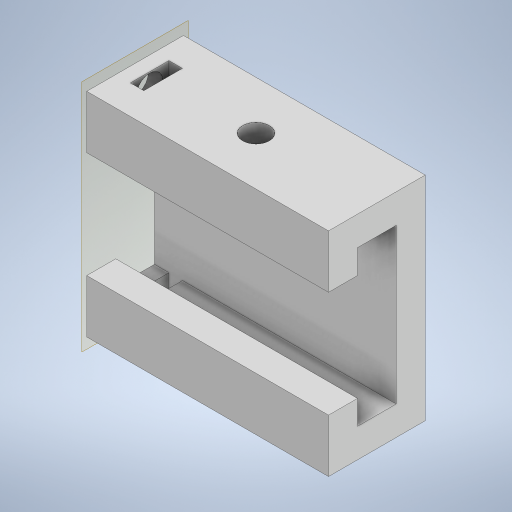
# Autodesk Inventor part: cuerpo_obj2
Saved by Autodesk Inventor 2023.2 (Build 272271030, 271C)
## iProperties
Created: 2023-02-25
Part Number: cuerpo_obj2
Material: Generic
Document SubType Name: Modeling
Designer: Cris Pat
Density: 1 g/cm^3
Appearance: Default
Author: Cris Pat
Autodesk Inventor part; units mm, degrees
ref_plane "XY Plane" through (0, 0, 0) normal (0, 0, 1) x (1, 0, 0)
sketch "Sketch1" plane through (0, 0, 0) normal (1, 0, 0) x (0, 1, 0)
  line L0 (11, 10) -> (11, 4)
  line L1 (11, 4) -> (16, 4)
  line L2 (16, 4) -> (16, -4)
  line L3 (16, -4) -> (-16, -4)
  line L4 (-16, -4) -> (-16, 4)
  line L5 (-16, 4) -> (-11, 4)
  line L6 (-11, 4) -> (-11, 10)
  line L7 (-11, 10) -> (-22, 10)
  line L8 (-22, 10) -> (-22, -10)
  line L9 (-22, -10) -> (22, -10)
  line L10 (22, -10) -> (22, 10)
  line L11 (22, 10) -> (11, 10)
  line L12 (11, 7) -> (-11, 7) construction
  line L13 (16, 0) -> (-16, 0) construction
  point P0 (0, 0)
  point P1 (-13.5, 4)
  point P2 (13.5, 4)
  point P3 (16.5, 10)
  point P4 (-16.5, 10)
  point P5 (22, 0)
  point P6 (0, -10)
  point P7 (0, 7)
  point P8 (0, 0)
  dimension "d0" = 22
  dimension "d1" = 32
  dimension "d2" = 6
  dimension "d3" = 14
  dimension "d4" = 44
  dimension "d5" = 20
  constraints: 28 end point, 12 midpoint, 10 perpendicular, 3 horizontal alignment, 3 point on line, 2 vertical alignment, 1 coincident, 1 vertical
  measures "d0" distance between parallel lines of L6 L0
  measures "d1" distance from line of L4 L13.start
  measures "d2" distance from line of point (-13.5, 4) L7
  measures "d3" distance between parallel lines of L7 L3
  measures "d4" distance between parallel lines of L8 L10
  measures "d5" distance between parallel lines of L7 L9
extrude "Extrusion1" add sketch "Sketch1" along normal mid plane 50
ref_plane "Work Plane1" through (0, 22, 0) normal (0, 1, 0) x (-1, 0, 0)
sketch "Sketch2" plane through (0, 22, 0) normal (0, 1, 0) x (-1, 0, 0)
  line L0 (25, 10) -> (-25, 10) construction
  line L1 (-25, -10) -> (-25, 10) construction
  line L2 (25, -10) -> (-25, -10) construction
  line L3 (25, 10) -> (25, -10) construction
  line L4 (-25, 0) -> (25, 0) construction
  circle A0 centre (0, 0) radius 2.75
  point P0 (0, 0)
  dimension "d9" = 5.5
  dimension "d10" = 25
  constraints: 3 midpoint, 2 end point, 1 centre point
  measures "d9" diameter of A0
  measures "d10" distance of L4.start A0.centre
extrude "Extrusion2" cut sketch "Sketch2" against normal up to surface (6 mm away)
sketch "Sketch3" plane through (0, 22, 0) normal (0, 1, 0) x (-1, 0, 0)
  line L0 (22, 4) -> (19.2, 4)
  line L1 (19.2, 4) -> (19.2, -4)
  line L2 (19.2, -4) -> (22, -4)
  line L3 (22, -4) -> (22, 4)
  line L4 (25, 10) -> (25, -10) construction
  point P0 (0, 0)
  point P1 (19.2, 0)
  dimension "d13" = 8
  dimension "d14" = 3
  dimension "d15" = 2.8
  constraints: 8 end point, 2 parallel, 1 horizontal, 1 horizontal alignment, 1 midpoint, 1 perpendicular
  measures "d13" distance between parallel lines of L0 L2
  measures "d14" distance between parallel lines of L3 L4
  measures "d15" distance between parallel lines of L1 L3
extrude "Extrusion3" cut sketch "Sketch3" against normal through all
ref_plane "Work Plane2" through (-25, 0, 0) normal (1, 0, 0) x (0, 1, 0)
sketch "Sketch4" plane through (-25, 0, 0) normal (1, 0, 0) x (0, 1, 0)
  circle A0 centre (19, 0) radius 2.75
  line L0 (0, -10) -> (0, 10) construction
  line L1 (22, -10) -> (-22, -10) construction
  circle A1 centre (-19, 0) radius 2.75
  point P0 (0, 0)
  point P1 (11, 10)
  point P2 (0, 0)
  dimension "d19" = 5.5
  dimension "d20" = 19
  constraints: 3 coincident, 2 centre point, 2 end point, 2 horizontal alignment, 2 midpoint, 1 symmetric about line, 1 vertical, 1 other
  measures "d19" diameter of A0
  measures "d20" distance of point (0, 0) A0.centre
extrude "Extrusion4" cut sketch "Sketch4" along normal blind 10
body "Solid1"
